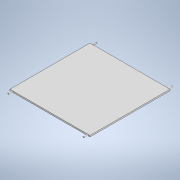
# Autodesk Inventor part: 01_10_Plataforma
Saved by Autodesk Inventor 2021 (Build 250183000, 183)
## iProperties
Created: 2021-06-25
Part Number: 01_10_Plataforma
Material: Genérico
Document SubType Name: Modeling
Designer: Almanzor
Density: 1 g/cm^3
Appearance: Valor por defecto
Author: Almanzor
Autodesk Inventor part; units mm, degrees
ref_plane "YZ Plane" through (0, 0, 0) normal (1, 0, 0) x (0, 1, 0)
ref_plane "XZ Plane" through (0, 0, 0) normal (0, 1, 0) x (-1, 0, 0)
ref_plane "XY Plane" through (0, 0, 0) normal (0, 0, 1) x (1, 0, 0)
sketch "Boceto1" plane through (0, 0, 0) normal (0, 1, 0) x (-1, 0, 0)
  line L0 (0, 0) -> (-1000, 0)
  line L1 (-1000, 0) -> (-1000, -1000)
  line L2 (-1000, -1000) -> (0, -1000)
  line L3 (0, -1000) -> (0, 0)
  dimension "d0" = 1000
  dimension "d1" = 1000
  constraints: 8 end point, 2 parallel, 1 horizontal, 1 perpendicular
  measures "d0" distance of L2.end L1.end
  measures "d1" distance of L0.end L1.end
extrude "Extrusión1" add sketch "Boceto1" along normal blind 17
sketch "Boceto2" plane through (0, 0, 0) normal (0, -1, 0) x (1, 0, 0)
  line L0 (286.7389, -300) -> (686.7389, -300)
  line L1 (0, 0) -> (1000, 0) projected
  line L2 (686.7389, -700) -> (286.7389, -700)
  line L3 (1000, -1000) -> (0, -1000) projected
  line L4 (686.7389, -300) -> (686.7389, -400)
  line L5 (286.7389, -300) -> (286.7389, -300)
  line L6 (286.7389, -300) -> (286.7389, -400)
  line L7 (286.7389, -700) -> (286.7389, -600)
  line L8 (686.7389, -700) -> (686.7389, -600)
  line L9 (286.7389, -400) -> (561.7389, -400)
  line L10 (286.7389, -600) -> (561.7389, -600)
  line L11 (561.7389, -600) -> (486.7389, -500)
  line L12 (486.7389, -500) -> (561.7389, -400)
  line L13 (686.7389, -400) -> (561.7389, -500)
  line L14 (561.7389, -500) -> (686.7389, -600)
  dimension "d4" = 300
  dimension "d5" = 300
  dimension "d6" = 100
  dimension "d7" = 100
  dimension "d8" = 100
  dimension "d9" = 100
  dimension "d10" = 200
  dimension "d11" = 400
  dimension "d12" = 400
  dimension "d13" = 275
  constraints: 26 end point, 5 horizontal, 4 vertical, 1 collinear
  measures "d4" distance between parallel lines of L1 L0
  measures "d5" distance between parallel lines of L3 L2
  measures "d6" distance of L0.end L4.end
  measures "d7" distance of L5.start L6.end
  measures "d8" distance of L2.end L7.end
  measures "d9" distance of L2.start L8.end
  measures "d10" distance of L8.end L4.end
  measures "d11" distance of L0.start L0.end
  measures "d12" distance of L2.start L2.end
  measures "d13" distance of L6.end L9.end
extrude "Extrusión2" cut sketch "Boceto2" against normal blind 1
sketch "Boceto3" plane through (0, 0, 0) normal (0, 0, 1) x (1, 0, 0)
  circle A0 centre (30, 8.5) radius 8.5
  line L0 (0, 0) -> (1000, 0) projected
  circle A1 centre (970, 8.5) radius 8.5
  line L1 (0, 0) -> (0, 17) projected
  line L2 (1000, 0) -> (1000, 17) projected
  dimension "d17" = 17
  dimension "d18" = 17
  dimension "d21" = 30
  dimension "d22" = 30
  constraints: 2 centre point, 2 tangent
  measures "d17" diameter of A0
  measures "d18" diameter of A1
  measures "d21" distance from line of L1 A0.centre
  measures "d22" distance from line of L2 A1.centre
extrude "Extrusión3" add sketch "Boceto3" along normal blind 50
sketch "Boceto5" plane through (1000, 0, -1000) normal (0, 0, -1) x (-1, 0, 0)
  circle A0 centre (30, 8.5) radius 8.5 projected
  circle A1 centre (30, 8.5) radius 8.5
  line L0 (0, 0) -> (0, 17) projected
  arc A2 (970, 0) -> (970, 17) centre (970, 8.5) ccw projected
  circle A3 centre (970, 8.5) radius 8.5
  line L1 (1000, 0) -> (1000, 17) projected
  line L2 (0, 0) -> (1000, 0) projected
  dimension "d23" = 30
  dimension "d24" = 30
  constraints: 2 centre point, 2 coincident, 1 tangent
  measures "d23" distance from line of L0 A1.centre
  measures "d24" distance from line of L1 A3.centre
extrude "Extrusión4" add sketch "Boceto5" along normal blind 50
